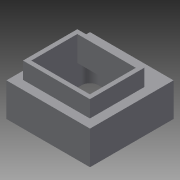
# Autodesk Inventor part: Case1
Saved by Autodesk Inventor 2014 (Build 180170000, 170)
## iProperties
Created: 2014-02-01
Part Number: Case1
Material: Generic
Document SubType Name: Modeling
Designer: Owner
Density: 1 g/cm^3
Appearance: Default
Author: Owner
Autodesk Inventor part; units mm, degrees
ref_plane "YZ Plane" through (0, 0, 0) normal (1, 0, 0) x (0, 1, 0)
ref_plane "XZ Plane" through (0, 0, 0) normal (0, 1, 0) x (-1, 0, 0)
ref_plane "XY Plane" through (0, 0, 0) normal (0, 0, 1) x (1, 0, 0)
sketch "Sketch1" plane through (0, 0, 0) normal (0, 1, 0) x (-1, 0, 0)
  line L0 (-50.8, 50.8) -> (50.8, 50.8)
  line L1 (50.8, 50.8) -> (50.8, -50.8)
  line L2 (50.8, -50.8) -> (-50.8, -50.8)
  line L3 (-50.8, -50.8) -> (-50.8, 50.8)
  line L4 (-63.5, 63.5) -> (63.5, 63.5)
  line L5 (63.5, 63.5) -> (63.5, -63.5)
  line L6 (63.5, -63.5) -> (-63.5, -63.5)
  line L7 (-63.5, -63.5) -> (-63.5, 63.5)
  point P0 (0, 0)
  dimension "d0" = 101.6
  dimension "d1" = 101.6
  dimension "d2" = 127
  dimension "d3" = 127
  dimension "d4" = 63.5
  dimension "d5" = 63.5
  dimension "d6" = 50.8
  dimension "d7" = 50.8
  constraints: 16 end point, 4 parallel, 2 horizontal, 2 perpendicular
  measures "d0" distance of L0.start L0.end
  measures "d1" distance of L0.end L1.end
  measures "d2" distance of L4.start L4.end
  measures "d3" distance of L6.end L4.start
  measures "d4" distance from line of point (0, 0) L4
  measures "d5" distance from line of point (0, 0) L5
  measures "d6" distance from line of point (0, 0) L0
  measures "d7" distance from line of point (0, 0) L1
extrude "Extrusion1" add sketch "Sketch1" against normal blind 38.1
fillet "Fillet1" radius 12.7 4 edges at (-50.8, -19.05, -50.8) (50.8, -19.05, -50.8) (-50.8, -19.05, 50.8) (50.8, -19.05, 50.8)
sketch "Sketch3" plane through (0, 0, 0) normal (0, 1, 0) x (1, 0, 0)
  line L0 (-63.5, 63.5) -> (63.5, 63.5)
  line L1 (63.5, 63.5) -> (63.5, -63.5)
  line L2 (63.5, -63.5) -> (-63.5, -63.5)
  line L3 (-63.5, -63.5) -> (-63.5, 63.5)
  point P0 (0, 0)
  constraints: 8 end point, 2 parallel, 1 horizontal, 1 perpendicular
extrude "Extrusion2" add sketch "Sketch3" along normal blind 12.7
sketch "Sketch4" plane through (0, 12.7, 0) normal (0, 1, 0) x (1, 0, 0)
  line L0 (63.5, -63.5) -> (63.5, 63.5) projected
  line L1 (63.5, 63.5) -> (-63.5, 63.5) projected
  circle A0 centre (38.1, 38.1) radius 3.175
  circle A1 centre (-69.85, 38.1) radius 3.175
  circle A2 centre (38.1, -69.85) radius 3.175
  circle A3 centre (-69.85, -69.85) radius 3.175
  point P0 (0, 0)
  dimension "d13" = 6.35
  dimension "d14" = 25.4
  dimension "d15" = 25.4
  dimension "d18" = 107.95
  dimension "d21" = 107.95
  constraints: 4 centre point, 1 horizontal, 1 vertical, 6 other
  measures "d13" diameter of A0
  measures "d14" distance from line of L1 A0.centre
  measures "d15" distance from line of L0 A0.centre
  measures "d18" distance of A0.centre A1.centre
  measures "d21" distance of A0.centre A2.centre
extrude "Extrusion3" cut sketch "Sketch4" against normal up to next
sketch "Sketch5" plane through (0, 12.7, 0) normal (0, 1, 0) x (1, 0, 0)
  circle A0 centre (50.8, -57.15) radius 3.175 projected
  circle A1 centre (38.1, 38.1) radius 3.175 projected
  circle A2 centre (-57.15, 50.8) radius 3.175 projected
  circle A3 centre (-57.15, -57.15) radius 3.175 projected
  circle A4 centre (-57.15, -57.15) radius 6.35
  circle A5 centre (-57.15, 50.8) radius 6.35
  circle A6 centre (38.1, 38.1) radius 6.35
  circle A7 centre (50.8, -57.15) radius 6.35
  point P0 (0, 0)
  dimension "d26" = 12.7
  dimension "d27" = 12.7
  dimension "d28" = 12.7
  dimension "d29" = 12.7
  constraints: 4 centre point, 4 coincident
  measures "d26" diameter of A7
  measures "d27" diameter of A6
  measures "d28" diameter of A5
  measures "d29" diameter of A4
extrude "Extrusion4" [suppressed]
sketch "Sketch6" plane through (0, 12.7, 0) normal (0, 1, 0) x (1, 0, 0)
  line L0 (-45.1827, 25.9215) -> (43.7173, 25.9215)
  line L1 (43.7173, 25.9215) -> (43.7173, -43.9285)
  line L2 (43.7173, -43.9285) -> (-45.1827, -43.9285)
  line L3 (-45.1827, -43.9285) -> (-45.1827, 25.9215)
  line L4 (-51.5327, 32.2715) -> (50.0673, 32.2715)
  line L5 (50.0673, 32.2715) -> (50.0673, -50.2785)
  line L6 (50.0673, -50.2785) -> (-51.5327, -50.2785)
  line L7 (-51.5327, -50.2785) -> (-51.5327, 32.2715)
  point P0 (0, 0)
  dimension "d32" = 69.85
  dimension "d33" = 88.9
  dimension "d36" = 6.35
  dimension "d37" = 6.35
  dimension "d38" = 6.35
  dimension "d39" = 6.35
  constraints: 16 end point, 4 parallel, 2 horizontal, 2 perpendicular
  measures "d32" distance of L0.end L1.end
  measures "d33" distance of L0.start L0.end
  measures "d36" distance between parallel lines of L0 L4
  measures "d37" distance between parallel lines of L7 L3
  measures "d38" distance between parallel lines of L6 L2
  measures "d39" distance between parallel lines of L5 L1
extrude "Extrusion5" add sketch "Sketch6" along normal blind 25.4
sketch "Sketch7" plane through (0, 12.7, 0) normal (0, 1, 0) x (1, 0, 0)
  line L0 (43.7173, -43.9285) -> (43.7173, 25.9215) projected
  line L1 (43.7173, 25.9215) -> (-45.1827, 25.9215) projected
  line L2 (-45.1827, 25.9215) -> (43.7173, 25.9215)
  line L3 (43.7173, 25.9215) -> (43.7173, -43.9285)
  line L4 (43.7173, -43.9285) -> (-45.1827, -43.9285)
  line L5 (-45.1827, -43.9285) -> (-45.1827, 25.9215)
  point P0 (0, 0)
  point P1 (63.5839, -35.7281)
  point P2 (63.5, 18.4248)
  constraints: 8 end point, 2 parallel, 1 horizontal, 1 perpendicular, 2 other
extrude "Extrusion6" cut sketch "Sketch7" against normal up to next
body "Solid1"
